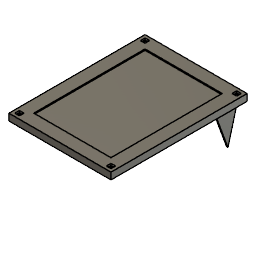
Ramecek_configurated (Autodesk Fusion 360 archive; units mm, degrees)
design "ramecekpokusdruhy"
part number: Foto 15×21
Autodesk Fusion 360 part; units mm, degrees
sketch "Sketch1" plane through (0, 0, 0) normal (0, 1, 0) x (1, 0, 0)
  line L0 (60, 85) -> (-60, -85) construction
  line L1 (-60, 85) -> (60, -85) construction
  line L2 (74, 104) -> (-74, 104)
  line L3 (-74, 104) -> (-74, -104)
  line L4 (-74, -104) -> (74, -104)
  line L5 (74, -104) -> (74, 104)
  line L6 (74, 104) -> (-74, -104) construction
  line L7 (-74, 104) -> (74, -104) construction
  line L8 (-76, 106) -> (-76, -106)
  line L9 (-76, -106) -> (76, -106)
  line L10 (76, -106) -> (76, 106)
  line L11 (76, 106) -> (-76, 106)
  line L12 (-85, 115) -> (-85, -115)
  line L13 (-85, -115) -> (85, -115)
  line L14 (85, -115) -> (85, 115)
  line L15 (85, 115) -> (-85, 115)
  dimension "d10" = 148
  dimension "d11" = 208
  dimension "d19" = 2
  dimension "d20" = 9
  constraint coincident L0 origin
  constraint coincident L1 origin
  constraint horizontal L2
  constraint perpendicular L2 L3
  constraint parallel L2 L4
  constraint parallel L3 L5
  constraint coincident L6 origin
  constraint coincident L7 origin
  measures "d10" distance of L3.end L4.end
  measures "d11" distance of L2.end L3.end
extrude "Extrude1" add sketch "Sketch1" along normal blind 10 contours L12 L13 L14 L15 makes body 1
extrude "Extrude2" add sketch "Sketch1" along normal blind 7.5 contours L8 L9 L10 L11 bodies 1
sketch "Sketch3" plane through (0, 0, 0) normal (0, 1, 0) x (1, 0, 0)
  line L0 (136.909, 72.3092) -> (272.909, 72.3092)
  line L1 (272.909, 72.3092) -> (272.909, -123.6908)
  line L2 (272.909, -123.6908) -> (136.909, -123.6908)
  line L3 (136.909, -123.6908) -> (136.909, 72.3092)
  line L4 (289.959, 89.3592) -> (289.959, -140.7408)
  line L5 (289.959, -140.7408) -> (119.859, -140.7408)
  line L6 (119.859, -140.7408) -> (119.859, 89.3592)
  line L7 (119.859, 89.3592) -> (289.959, 89.3592)
  line L8 (294.959, -145.7408) -> (114.859, -145.7408)
  line L9 (114.859, -145.7408) -> (114.859, 94.3592)
  line L10 (114.859, 94.3592) -> (294.959, 94.3592)
  line L11 (294.959, 94.3592) -> (294.959, -145.7408)
  dimension "d16" = 136
  dimension "d17" = 196
  dimension "d18" = -17.05
  dimension "d21" = -5
  constraint horizontal L0
  constraint vertical L1
  constraint horizontal L2
  constraint vertical L3
  measures "d16" distance of L0.start L0.end
  measures "d17" distance of L0.start L2.end
extrude "Extrude3" add sketch "Sketch3" along normal blind 12 separate body contours L8 L9 L10 L11 makes body 2
extrude "Extrude4" add sketch "Sketch3" along normal blind 2 contours L4 L5 L6 L7 bodies 2
sketch "Sketch4" plane through (0, 10, 0) normal (0, 1, 0) x (-1, 0, 0)
  line L0 (76, -106) -> (-76, -106)
  line L1 (-76, -106) -> (-76, 106)
  line L2 (-76, 106) -> (76, 106)
  line L3 (76, 106) -> (76, -106)
  line L4 (-85, -115) -> (85, -115)
  line L5 (85, -115) -> (85, 115)
  line L6 (85, 115) -> (-85, 115)
  line L7 (-85, 115) -> (-85, -115)
  line L8 (78.25, -113.25) -> (83.25, -113.25)
  line L9 (83.25, -113.25) -> (83.25, -108.25)
  line L10 (83.25, -108.25) -> (78.25, -108.25)
  line L11 (78.25, -108.25) -> (78.25, -113.25)
  line L12 (78.25, -113.25) -> (83.25, -108.25) construction
  line L13 (83.25, -113.25) -> (78.25, -108.25) construction
  line L14 (0, -121.5702) -> (0, -108.4298)
  line L15 (93.3817, 0) -> (76.6183, 0)
  line L16 (-78.25, -108.25) -> (-78.25, -113.25)
  line L17 (-78.25, -113.25) -> (-83.25, -113.25)
  line L18 (-83.25, -113.25) -> (-83.25, -108.25)
  line L19 (-83.25, -108.25) -> (-78.25, -108.25)
  line L20 (78.25, 113.25) -> (83.25, 113.25)
  line L21 (83.25, 113.25) -> (83.25, 108.25)
  line L22 (83.25, 108.25) -> (78.25, 108.25)
  line L23 (78.25, 108.25) -> (78.25, 113.25)
  line L24 (-78.25, 108.25) -> (-78.25, 113.25)
  line L25 (-78.25, 113.25) -> (-83.25, 113.25)
  line L26 (-83.25, 113.25) -> (-83.25, 108.25)
  line L27 (-83.25, 108.25) -> (-78.25, 108.25)
  point P0 (80.75, -110.75)
  dimension "d27" = 5
  dimension "d83" = 1.75
  dimension "d84" = 1.75
  constraint horizontal L8
  constraint perpendicular L8 L9
  constraint parallel L8 L10
  constraint parallel L9 L11
  constraint coincident L12 P0
  constraint coincident L13 P0
  constraint perpendicular L0 L14
  constraint midpoint L4 L14
  constraint perpendicular L3 L15
  constraint midpoint L5 L15
  constraint equal L8 L9
  constraint symmetric L8.start L14 L16.end
  constraint symmetric L8.end L14 L17.end
  constraint symmetric L9.end L14 L18.end
  constraint symmetric L10.end L14 L16.start
  constraint symmetric L8.start L15 L20.start
  constraint symmetric L8.end L15 L20.end
  constraint symmetric L9.end L15 L21.end
  constraint symmetric L10.end L15 L22.end
  constraint symmetric L15 L16.start L24.start
  constraint symmetric L15 L16.end L24.end
  constraint symmetric L15 L17.end L25.end
  constraint symmetric L15 L18.end L26.end
  measures "d27" distance of L9 L11
  measures "d83" distance of L5 L9
  measures "d84" distance of L4 L8
copy_body "Body->Comp1" bodies 1 removing the originals makes body 3 in component "Spodní část rámečku"
copy_body "Body->Comp2" bodies 2 removing the originals makes body 4 in component "Horní část rámečku"
extrude "Extrude1'" cut sketch "Sketch4" against normal blind 1.9 contours L8 L9 L10 L11 | L16 L17 L18 L19 | L20 L21 L22 L23 | L24 L25 L26 L27 bodies 3 in component "Spodní část rámečku"
sketch "Sketch7" plane through (0, 0, 0) normal (0, 1, 0) x (1, 0, 0)
  line L0 (115.4319, 0.7999) -> (188.2572, 0.7999)
  line L1 (122.9878, 0.7999) -> (122.9878, 40.7999)
  line L2 (122.9878, 0.7999) -> (186.287, 23.839)
  line L3 (122.9878, 0.7999) -> (201, 0.7999) construction
  line L4 (122.9878, 40.7999) -> (186.287, 23.839)
  line L5 (122.9878, 40.7999) -> (117.9878, 40.7999)
  line L6 (117.9878, 40.7999) -> (117.9878, 0.7999)
  line L7 (117.9878, 0.7999) -> (122.9878, 0.7999)
  line L8 (122.9878, 0.7999) -> (122.9878, 40.7999)
  line L9 (122.9878, 40.7999) -> (185, 40.7999)
  dimension "d36" = 40
  dimension "d38" = 20
  dimension "d39" = 5
  dimension "d40" = 40
  dimension "d65" = 15
  constraint horizontal L0
  constraint coincident L0 L1.start
  constraint perpendicular L0 L1
  constraint horizontal L3
  constraint horizontal L5
  constraint vertical L6
  constraint horizontal L7
  constraint vertical L8
  constraint perpendicular L1 L9
  measures "d36" distance of L1.start L1.end
  measures "d38" angle of L2 L3
  measures "d39" distance of L1.end L5.end
  measures "d40" distance of L1.end L1.start
  measures "d65" angle of L4 L9
extrude "Extrude5" add sketch "Sketch7" along normal blind 2.4 separate body makes body 5
move_body "Move1" bodies 3 to x (-1, 0, 0) y (0, -1, 0) z (0, 0, 1) at (-170, 20, 0) in component "Spodní část rámečku"
move_body "Move1'" bodies 4 to x (1, 0, 0) y (0, 1, 0) z (0, 0, 1) at (42.7114, 0, -13.3808) in component "Horní část rámečku"
sketch "Sketch9" plane through (0, 20, 0) normal (0, 1, 0) x (-1, 0, 0)
  line L0 (244, 104) -> (244, -104)
  line L1 (244, -104) -> (96, -104)
  line L2 (96, -104) -> (96, 104)
  line L3 (96, 104) -> (244, 104)
  line L4 (85, -115) -> (255, -115)
  line L5 (255, -115) -> (255, 115)
  line L6 (255, 115) -> (85, 115)
  line L7 (85, 115) -> (85, -115)
  line L8 (89.25, -72.5) -> (91.75, -72.5)
  line L9 (91.75, -72.5) -> (91.75, -112.6)
  line L10 (91.75, -112.6) -> (89.25, -112.6)
  line L11 (89.25, -112.6) -> (89.25, -72.5)
  line L12 (85, -72.5) -> (96, -72.5)
  line L13 (90.5, -70.5305) -> (90.5, -74.4695)
  line L14 (170, 115) -> (170, 93)
  line L15 (250.75, -112.6) -> (250.75, -72.5)
  line L16 (250.75, -72.5) -> (248.25, -72.5)
  line L17 (248.25, -72.5) -> (248.25, -112.6)
  line L18 (248.25, -112.6) -> (250.75, -112.6)
  line L19 (87.4, 110.75) -> (127.5, 110.75)
  line L20 (127.5, 110.75) -> (127.5, 108.25)
  line L21 (127.5, 108.25) -> (87.4, 108.25)
  line L22 (87.4, 108.25) -> (87.4, 110.75)
  line L23 (123.7485, 109.5) -> (131.2515, 109.5)
  line L24 (76, 0) -> (116, 0)
  line L25 (87.4, -110.75) -> (127.5, -110.75)
  line L26 (127.5, -110.75) -> (127.5, -108.25)
  line L27 (127.5, -108.25) -> (87.4, -108.25)
  line L28 (87.4, -108.25) -> (87.4, -110.75)
  point P0 (170, 104)
  dimension "d44" = 2.5
  dimension "d45" = 40.1
  dimension "d46" = 2.4
  dimension "d55" = 40.1
  dimension "d56" = 2.5
  dimension "d57" = 2.4
  constraint horizontal L8
  constraint vertical L9
  constraint horizontal L10
  constraint vertical L11
  constraint coincident L7 L12.start
  constraint coincident L2 L12.end
  constraint perpendicular L2 L12
  constraint perpendicular L12 L13
  constraint midpoint L12 L13
  constraint midpoint L8 L12
  constraint perpendicular L3 L14
  constraint midpoint L3 L14
  constraint symmetric L8.start L14 L15.end
  constraint symmetric L8.end L14 L16.end
  constraint symmetric L9.end L14 L17.end
  constraint symmetric L10.end L14 L15.start
  constraint horizontal L19
  constraint vertical L20
  constraint horizontal L21
  constraint vertical L22
  constraint coincident L6 L14.start
  constraint midpoint L14 P0
  constraint perpendicular L14 L23
  constraint symmetric L14.start P0 L23
  constraint midpoint L20 L23
  constraint horizontal L24
  constraint midpoint L2 L24
  constraint symmetric L19.start L24 L25.start
  constraint symmetric L19.end L24 L25.end
  constraint symmetric L20.end L24 L26.end
  constraint symmetric L21.end L24 L27.end
  measures "d44" distance of L8.start L8.end
  measures "d45" distance of L8.start L10.end
  measures "d46" distance of L4 L10
  measures "d55" distance of L19.start L19.end
  measures "d56" distance of L19.start L21.end
  measures "d57" distance of L7 L22
extrude "Extrude2'" cut sketch "Sketch9" against normal blind 5.1 contours L8 L9 L11 L12 L27 | L9 L25 L26 L27 | L9 L11 L25 L27 | L9 L10 L11 L25 | L11 L25 L27 L28 | L15 L16 L17 L18 | L19 L20 L21 L22 bodies 3 in component "Spodní část rámečku"
sketch "Sketch10" plane through (0, 0, 0) normal (0, 1, 0) x (1, 0, 0)
  line L0 (167.5841, -53.6023) -> (379.3841, -53.6023)
  line L1 (379.3841, -53.6023) -> (379.3841, -205.4023)
  line L2 (379.3841, -205.4023) -> (167.5841, -205.4023)
  line L3 (167.5841, -205.4023) -> (167.5841, -53.6023)
  dimension "d50" = 211.8
  dimension "d51" = 151.8
  constraint horizontal L0
  constraint vertical L1
  constraint horizontal L2
  constraint vertical L3
  measures "d50" distance of L0.start L0.end
  measures "d51" distance of L0.start L2.end
extrude "Extrude6" add sketch "Sketch10" along normal blind 1.4 separate body makes body 6
sketch "Sketch11" plane through (197.909, 2, 43.7408) normal (0, 1, 0) x (1, 0, 0)
  line L0 (117.7114, -66.5692) -> (-18.2886, -66.5692)
  line L1 (-18.2886, -66.5692) -> (-18.2886, 129.4308)
  line L2 (-18.2886, 129.4308) -> (117.7114, 129.4308)
  line L3 (117.7114, 129.4308) -> (117.7114, -66.5692)
  line L4 (-35.3386, 146.4808) -> (-35.3386, -83.6192)
  line L5 (-35.3386, -83.6192) -> (134.7614, -83.6192)
  line L6 (134.7614, -83.6192) -> (134.7614, 146.4808)
  line L7 (134.7614, 146.4808) -> (-35.3386, 146.4808)
  line L8 (-28.4886, -76.7692) -> (-33.4886, -76.7692)
  line L9 (-33.4886, -76.7692) -> (-33.4886, -81.7692)
  line L10 (-33.4886, -81.7692) -> (-28.4886, -81.7692)
  line L11 (-28.4886, -81.7692) -> (-28.4886, -76.7692)
  line L12 (-28.4886, -76.7692) -> (-33.4886, -81.7692) construction
  line L13 (-33.4886, -76.7692) -> (-28.4886, -81.7692) construction
  line L14 (49.7114, -57.4623) -> (49.7114, -75.6762)
  line L15 (-40.1147, 31.4308) -> (3.5375, 31.4308)
  line L16 (127.9114, -76.7692) -> (132.9114, -76.7692)
  line L17 (132.9114, -76.7692) -> (132.9114, -81.7692)
  line L18 (132.9114, -81.7692) -> (127.9114, -81.7692)
  line L19 (127.9114, -81.7692) -> (127.9114, -76.7692)
  line L20 (-28.4886, 139.6308) -> (-33.4886, 139.6308)
  line L21 (-33.4886, 139.6308) -> (-33.4886, 144.6308)
  line L22 (-33.4886, 144.6308) -> (-28.4886, 144.6308)
  line L23 (-28.4886, 144.6308) -> (-28.4886, 139.6308)
  line L24 (127.9114, 144.6308) -> (127.9114, 139.6308)
  line L25 (127.9114, 139.6308) -> (132.9114, 139.6308)
  line L26 (132.9114, 139.6308) -> (132.9114, 144.6308)
  line L27 (132.9114, 144.6308) -> (127.9114, 144.6308)
  point P0 (-30.9886, -79.2692)
  dimension "d58" = 5
  dimension "d59" = 5
  dimension "d61" = 1.85
  dimension "d62" = 1.85
  constraint horizontal L8
  constraint perpendicular L8 L9
  constraint parallel L8 L10
  constraint parallel L9 L11
  constraint coincident L12 P0
  constraint coincident L13 P0
  constraint perpendicular L0 L14
  constraint midpoint L0 L14
  constraint horizontal L15
  constraint midpoint L1 L15
  constraint symmetric L8.start L14 L16.start
  constraint symmetric L8.end L14 L16.end
  constraint symmetric L9.end L14 L17.end
  constraint symmetric L10.end L14 L18.end
  constraint symmetric L8.start L15 L20.start
  constraint symmetric L8.end L15 L20.end
  constraint symmetric L9.end L15 L21.end
  constraint symmetric L10.end L15 L22.end
  constraint symmetric L15 L16.start L24.end
  constraint symmetric L15 L16.end L25.end
  constraint symmetric L15 L17.end L26.end
  constraint symmetric L15 L18.end L24.start
  measures "d58" distance of L9.end L10.end
  measures "d59" distance of L8.end L9.end
  measures "d61" distance of L5 L10
  measures "d62" distance of L4 L9
extrude "Extrude2''" cut sketch "Sketch11" against normal blind 5 contours L8 L9 L10 L11 | L16 L17 L18 L19 | L20 L21 L22 L23 | L24 L25 L26 L27 bodies 4 in component "Horní část rámečku"
move_body "Move2" bodies 3 to x (-1, 0, 0) y (0, -1, 0) z (0, 0, 1) at (-170, 40, 0) in component "Spodní část rámečku"
copy_body "Body->Comp3" bodies 5 removing the originals makes body 7 in component "Noha rámečku"
copy_body "Body->Comp4" bodies 6 removing the originals makes body 8 in component "Deska horizontálně"
fillet "Fillet1" radius 1.5 4 edges at (328.3204, 0, -100.89) (330.8204, 0, -98.39) (328.3204, 0, -95.89) (325.8204, 0, -98.39) on bodies 4 in component "Horní část rámečku"
fillet "Fillet1" radius 1.5 4 edges at (166.9204, 0, -100.89) (169.4204, 0, -98.39) (166.9204, 0, -95.89) (164.4204, 0, -98.39) on bodies 4 in component "Horní část rámečku"
fillet "Fillet1" radius 1.5 4 edges at (166.9204, 0, 120.51) (169.4204, 0, 123.01) (166.9204, 0, 125.51) (164.4204, 0, 123.01) on bodies 4 in component "Horní část rámečku"
fillet "Fillet1" radius 1.5 4 edges at (328.3204, 0, 120.51) (330.8204, 0, 123.01) (328.3204, 0, 125.51) (325.8204, 0, 123.01) on bodies 4 in component "Horní část rámečku"
component "Spodní část rámečku" placed x (1, 0, 0) y (0, 1, 0) z (0, 0, 1) at (0, 0, 0)
component "Horní část rámečku" placed x (-1, 0, 0) y (0, -1, 0) z (0, 0, 1) at (247.6704, 32.1, -12.26)
component "Noha rámečku" placed x (0, -1, 0) y (1, 0, 0) z (0, 0, 1) at (-80.7, 143.0878, -71.8001)
component "Deska horizontálně" placed x (0, 0, 1) y (0, 1, 0) z (-1, 0, 0) at (129.4023, 27.7, -273.3841)
component "Noha rámečku" placed x (0, -1, 0) y (1, 0, 0) z (0, 0, 1) at (78.3, 143.0878, -71.7501)
equation "foto_sirka = 150 mm"
equation "vule = 2 mm"
equation "foto_vyska = 210 mm"
equation "ram_sirka = 9 mm"
equation "ram_hloubka = 10 mm"
equation "d10 = foto_sirka - vule"
equation "d11 = foto_vyska - vule"
equation "d16 = foto_sirka - spadavka"
equation "d17 = foto_vyska - spadavka"
equation "d18 = -( ram_sirka + vule / 2 + spadavka / 2 + 0.05 mm )"
equation "d19 = vule"
equation "d20 = ram_sirka"
equation "d22 = ram_hloubka + vule"
equation "d24 = vule"
equation "dira = 5 mm"
equation "d27 = dira"
equation "d34 = -4.1 mm + 2.2 mm"
equation "d36 = noha_výška"
equation "d40 = noha_výška"
equation "d45 = noha_výška + 0.1 mm"
equation "spadavka = 14 mm"
equation "d50 = foto_vyska + 1.8 mm"
equation "d51 = foto_sirka + 1.8 mm"
equation "d55 = noha_výška + 0.1 mm"
equation "d58 = dira"
equation "d59 = dira"
equation "noha_výška = 40 mm"
named bodies: "Noha rámečku", "Deska horizontálně"
